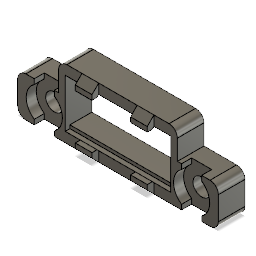
FSR_circuit_mount (Autodesk Fusion 360 design; units mm, degrees)
Autodesk Fusion 360 part; units mm, degrees
sketch "Sketch1" plane through (0, 0, 0) normal (0, 0, 1) x (1, 0, 0)
  line L0 (0, 0) -> (12, 0)
  line L1 (12, 0) -> (12, 60)
  line L2 (12, 60) -> (0, 60)
  line L3 (0, 0) -> (0, 12.25)
  line L4 (0, 12.25) -> (-8.5, 12.25)
  line L5 (-8.5, 12.25) -> (-8.5, 47.75)
  line L6 (-8.5, 47.75) -> (0, 47.75)
  line L7 (0, 47.75) -> (0, 60)
  line L8 (-5.5, 45.75) -> (9, 45.75)
  line L9 (9, 45.75) -> (9, 14.25)
  line L10 (9, 14.25) -> (-5.5, 14.25)
  line L11 (-5.5, 14.25) -> (-5.5, 45.75)
  line L12 (9, 30) -> (12, 30) construction
  line L13 (-8.5, 30) -> (-5.5, 30) construction
  line L14 (-2.6313, 47.75) -> (-2.6313, 45.75) construction
  line L15 (12, 30) -> (6, 30) construction
  line L16 (6, 30) -> (6, 8) construction
  line L17 (6, 30) -> (6, 52) construction
  line L18 (6, 60) -> (6, 52) construction
  circle A0 centre (6, 52) radius 2.6
  circle A1 centre (6, 8) radius 2.6
  circle A2 centre (6, 52) radius 5.4
  circle A3 centre (6, 8) radius 5.4
  line L19 (-8.0045, 55) -> (29, 55)
  line L20 (29, 55) -> (29, 49)
  line L21 (29, 49) -> (-8.0045, 49)
  line L22 (-8.0045, 49) -> (-8.0045, 55)
  line L23 (6, 52) -> (-8.0045, 52) construction
  line L24 (-6, 11) -> (49, 11)
  line L25 (49, 11) -> (49, 5)
  line L26 (49, 5) -> (-6, 5)
  line L27 (-6, 5) -> (-6, 11)
  line L28 (6, 8) -> (-6, 8) construction
  dimension "d1" = 60
  dimension "d2" = 12
  dimension "d3" = 31.5
  dimension "d4" = 14.5
  dimension "d5" = 2
  dimension "d6" = 8
  dimension "d7" = 5.2
  dimension "d8" = 10.8
  dimension "d9" = 3
  dimension "d10" = 6
  dimension "d11" = 6
  measures "d2" distance of L0.start
  measures "d7" diameter of A1
  measures "d8" diameter of A2
extrude "Extrude1" add sketch "Sketch1" against normal blind 8 contours L0 L1 L3 A3 L26 | L3 A3 L24 L26 | L1 A3 L24 L26 | L1 L3 L4 L5 L6 L7 A2 A3 L21 L24 | A3 L26 | A3 L24 L26 | A3 L24 | L1 A2 L19 L21 | L1 L2 L7 A2 L19 | A2 L19 L21 | A2 L21 | A2 L19 | L7 A2 L19 L21 | L8 L9 L10 L11
extrude "Extrude2" cut sketch "Sketch1" against normal blind 3 contours L3 A3 L24 L26 | L1 A3 L24 L26 | A3 L26 | A3 L24 L26 | A3 L24 | L1 A2 L19 L21 | A2 L19 L21 | A2 L21 | A2 L19 | L7 A2 L19 L21
extrude "Extrude3" cut sketch "Sketch1" against normal blind 1.4 contours L8 L9 L10 L11
fillet "Fillet1" radius 2.5 6 edges at (0, 60, -4) (12, 60, -4) (0, 0, -4) (12, 0, -4) (-8.5, 12.25, -4) (-8.5, 47.75, -4)
sketch "Sketch2" plane through (0, 0, -1.4) normal (0, 0, 1) x (1, 0, 0)
  line L0 (-5.5, 14.25) -> (9, 14.25)
  line L1 (9, 14.25) -> (9, 45.75)
  line L2 (9, 45.75) -> (-5.5, 45.75)
  line L3 (-5.5, 45.75) -> (-5.5, 14.25)
  line L4 (-4.5, 45.75) -> (8, 45.75)
  line L5 (8, 45.75) -> (8, 14.25)
  line L6 (8, 14.25) -> (-4.5, 14.25)
  line L7 (-4.5, 14.25) -> (-4.5, 45.75)
  line L8 (-4.5, 30) -> (-5.5, 30) construction
  line L9 (8, 30) -> (9, 30) construction
  dimension "d19" = 12.5
  dimension "d20" = 31.5
extrude "Extrude4" cut sketch "Sketch2" against normal blind 29 contours L0 L2 L4 L5 L6 L7
sketch "Sketch3" plane through (0, 12.25, 0) normal (0, -1, 0) x (1, 0, 0)
  line L0 (-6, 0) -> (-6, -8)
  line L1 (0, -8) -> (0, 0)
  line L2 (0, 0) -> (-6, 0)
  line L3 (-8.5, 0) -> (-8.5, 2)
  line L4 (-8.5, 2) -> (-5, 2)
  line L5 (-5, 2) -> (-5, 0.5)
  line L6 (-5, 0.5) -> (-5.5, 0)
  line L7 (-5.5, 0) -> (-8.5, 0)
  line L8 (12, 0) -> (12, -8)
  line L9 (12, 0) -> (12, 2)
  line L10 (12, 2) -> (8.5, 2)
  line L11 (8.5, 2) -> (8.5, 0.5)
  line L12 (8.5, 0.5) -> (9, 0)
  line L13 (9, 0) -> (12, 0)
  line L14 (-6, -8) -> (0, -8)
  dimension "d23" = 3.5
  dimension "d26" = 3
  dimension "d27" = 1.5
  dimension "d28" = 2
  dimension "d29" = 3.5
  dimension "d30" = 2
  dimension "d31" = 1.5
  dimension "d41" = 3
extrude "Extrude5" add sketch "Sketch3" against normal blind 64 contours L2 L3 L4 L5 L6 L7 | L9 L10 L11 L12 L13
sketch "Sketch4" plane through (0, 0, 2) normal (0, 0, 1) x (1, 0, 0)
  line L0 (-8.5, 12.25) -> (-5, 12.25)
  line L1 (-5, 12.25) -> (-5, 76.25)
  line L2 (-5, 76.25) -> (-8.5, 76.25)
  line L3 (-8.5, 76.25) -> (-8.5, 12.25)
  line L4 (-43, 87) -> (35, 87)
  line L5 (35, 87) -> (35, 40.75)
  line L6 (35, 40.75) -> (-43, 40.75)
  line L7 (-43, 40.75) -> (-43, 87)
  line L8 (-33, 35.75) -> (44, 35.75)
  line L9 (44, 35.75) -> (44, 24.25)
  line L10 (44, 24.25) -> (-33, 24.25)
  line L11 (-33, 24.25) -> (-33, 35.75)
  line L12 (-33, 19.25) -> (46, 19.25)
  line L13 (46, 19.25) -> (46, 6)
  line L14 (46, 6) -> (-33, 6)
  line L15 (-33, 6) -> (-33, 19.25)
  line L16 (-23, 40.75) -> (-23, 35.75) construction
  line L17 (-27, 24.25) -> (-27, 19.25) construction
  line L18 (9, 14.25) -> (-5.5, 14.25)
  line L19 (-5.0331, 19.25) -> (-5.0331, 14.25) construction
  line L20 (-5.5, 45.75) -> (9, 45.75)
  line L21 (-6, 40.75) -> (-6, 45.75) construction
  dimension "d36" = 5
  dimension "d37" = 5
  dimension "d38" = 5
  dimension "d39" = 5
  measures "d37" distance of origin
extrude "Extrude6" cut sketch "Sketch4" against normal blind 2 contours L0 L1 L3 L12 | L0 L1 L3 L12 L13 L14 L15 | L3 L8 L10 L11 | L1 L3 L8 L10 | L1 L8 L9 L10 | L1 L2 L3 L4 L5 L6 L7 | L1 L2 L3 L6
chamfer "Chamfer1" distance 2 angle 45 4 edges at (12, 38.25, 2) (-8.5, 38.25, 2) (-8.5, 21.75, 2) (12, 21.75, 2)
move_body "Move1" bodies 1 to x (0, -1, 0) y (1, 0, 0) z (0, 0, 1) at (-8.5, -8.5, 0)
